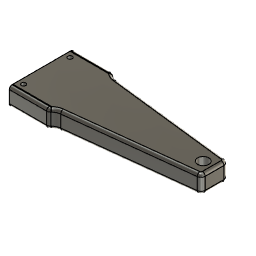
torsionEndPiece_vFINAL v4 (Autodesk Fusion 360 design; units mm, degrees)
Autodesk Fusion 360 part; units mm, degrees
sketch "Sketch1" plane through (0, 0, 0) normal (0, 0, 1) x (1, 0, 0)
  line L0 (0, 0) -> (0, 16)
  line L1 (86.957, 0) -> (0, 0)
  line L2 (0, 16) -> (21.957, 16)
  line L3 (86.957, 0) -> (86.957, 5)
  line L4 (86.957, 5) -> (21.957, 16)
  line L5 (86.957, -5) -> (21.957, -16)
  line L6 (0, -16) -> (21.957, -16)
  line L7 (86.957, 0) -> (86.957, -5)
  line L8 (0, 0) -> (0, -16)
  line L9 (86.957, 5) -> (96.957, 5)
  line L10 (96.957, 5) -> (96.957, -5)
  line L11 (96.957, -5) -> (86.957, -5)
  line L12 (86.957, -5) -> (86.957, 5)
  line L13 (21.957, 16) -> (96.957, 5)
  line L14 (96.957, -5) -> (21.957, -16)
  line L15 (96.957, 5) -> (96.957, 7.35)
  line L16 (96.957, -5) -> (96.957, -7.35)
  line L17 (96.957, 7.35) -> (21.957, 16)
  line L18 (96.957, -7.35) -> (21.957, -16)
  dimension "d1" = 16
  dimension "d20" = 21.957
  dimension "d47" = 65
  dimension "d48" = 5
  dimension "d49" = 10
  dimension "d56" = 2.35
  dimension "d57" = 2.35
  constraint coincident L0.start L1.end
  constraint vertical L0
  constraint perpendicular L0 L1
  constraint perpendicular L0 L2
  constraint perpendicular L1 L3
  constraint symmetric L0.start L1 L8.start
  constraint symmetric L0.end L1 L6.start
  constraint symmetric L3.start L1 L7.start
  constraint symmetric L1 L2.end L5.end
  constraint symmetric L1 L3.end L5.start
  constraint horizontal L9
  constraint vertical L10
  constraint horizontal L11
  constraint vertical L12
  constraint perpendicular L9 L15
  constraint perpendicular L11 L16
  measures "d1" distance of L0.start L0.end
  measures "d20" distance of L0.end L2.end
  measures "d47" horizontal distance of L2.end L3.end
  measures "d48" distance of L1.start L3.end
  measures "d49" distance of L3.end L9.end
  measures "d56" distance of L9.end L15.end
  measures "d57" distance of L10.end L16.end
extrude "Extrude1" add sketch "Sketch1" along normal blind 10 contours L0 L1 L2 L3 L4 L12 | L1 L5 L6 L7 L8 L12
sketch "Sketch2" plane through (0, 0, 0) normal (0, 0, 1) x (1, 0, 0)
  line L0 (0, 16) -> (0, -16)
sketch "Sketch3" plane through (0, 0, 0) normal (-1, 0, 0) x (0, -1, 0)
  line L0 (-16, 0) -> (16, 0)
  line L1 (16, 10) -> (-16, 10)
  line L2 (-16, 8) -> (-11, 8)
  line L3 (-7, 8) -> (-2, 8)
  line L4 (2, 8) -> (7.0009, 8)
  line L5 (-16, 10) -> (-16, 0)
  line L6 (7.0009, 8) -> (7.0009, 2)
  line L7 (7.0009, 2) -> (2, 2)
  line L8 (2, 2) -> (2, 8)
  line L9 (-2, 8) -> (-2, 2)
  line L10 (-2, 2) -> (-7, 2)
  line L11 (-7, 2) -> (-7, 8)
  line L12 (-11, 8) -> (-11, 2)
  line L13 (-11, 2) -> (-16, 2)
  line L14 (16, 8) -> (11, 8)
  line L15 (11, 8) -> (11, 2)
  line L16 (11, 2) -> (16, 2)
  line L17 (16, 2) -> (16, 8)
  dimension "d13" = 5
  dimension "d14" = 5
  dimension "d34" = 4
  dimension "d35" = 4
  constraint perpendicular L4 L6
  constraint perpendicular L6 L7
  constraint perpendicular L3 L9
  constraint perpendicular L9 L10
  constraint perpendicular L2 L12
  constraint coincident L5 L13.end
  constraint perpendicular L5 L13
  constraint horizontal L14
  constraint perpendicular L14 L15
  constraint perpendicular L15 L16
  constraint perpendicular L14 L17
  measures "d13" distance of L2.end L2.start
  measures "d14" distance of L3.start L3.end
  measures "d34" distance of L8 L9
  measures "d35" distance of L11 L12
extrude "Extrude2" cut sketch "Sketch3" against normal blind 20
sketch "Sketch5" plane through (0, 0, 10) normal (0, 0, 1) x (-1, 0, 0)
  line L0 (0, -16) -> (0, 16)
  line L1 (0, 16) -> (-21.957, 16)
  line L2 (-21.957, 16) -> (-86.957, 5)
  line L3 (-86.957, 5) -> (-86.957, -5)
  line L4 (-86.957, -5) -> (-21.957, -16)
  line L5 (-21.957, -16) -> (0, -16)
  circle A0 centre (-3, -13) radius 1
  circle A1 centre (-3, 13) radius 1
  dimension "d24" = 2
  dimension "d25" = 2
  dimension "d26" = 3
  dimension "d27" = 3
  dimension "d28" = 3
  dimension "d29" = 3
  measures "d24" diameter of A0
  measures "d25" diameter of A1
  measures "d26" distance of L0 A0.centre
  measures "d27" distance of L5 A0.centre
  measures "d28" distance of L0 A1.centre
  measures "d29" distance of L1 A1.centre
sketch "Sketch6" plane through (0, 0, 0) normal (-1, 0, 0) x (0, -1, 0)
  line L0 (-11, 2) -> (-16, 2)
  line L1 (-16, 2) -> (-16, 0)
  line L2 (-16, 0) -> (16, 0)
  line L3 (16, 0) -> (16, 2)
  line L4 (16, 2) -> (11, 2)
  line L5 (11, 2) -> (11, 8)
  line L6 (11, 8) -> (16, 8)
  line L7 (16, 8) -> (16, 10)
  line L8 (16, 10) -> (-16, 10)
  line L9 (-16, 10) -> (-16, 8)
  line L10 (-16, 8) -> (-11, 8)
  line L11 (-11, 8) -> (-11, 2)
  line L12 (-2, 8) -> (-2, 2)
  line L13 (-2, 2) -> (-7, 2)
  line L14 (-7, 2) -> (-7, 8)
  line L15 (-7, 8) -> (-2, 8)
  line L16 (7.0009, 8) -> (7.0009, 2)
  line L17 (7.0009, 2) -> (2, 2)
  line L18 (2, 2) -> (2, 8)
  line L19 (2, 8) -> (7.0009, 8)
  line L20 (16, 0) -> (18, 0)
  line L21 (18, 0) -> (18, 10)
  line L22 (18, 10) -> (16, 10)
  line L23 (16, 2) -> (16, 8)
  line L24 (16, 2) -> (16, 0)
  line L25 (16, 8) -> (16, 10)
  line L26 (-16, 0) -> (-18, 0)
  line L27 (-18, 0) -> (-18, 10)
  line L28 (-18, 10) -> (-16, 10)
  line L29 (-16, 8) -> (-16, 2)
  line L30 (-16, 2) -> (-16, 0)
  line L31 (-16, 8) -> (-16, 10)
  dimension "d36" = 2
  dimension "d37" = 10
  constraint coincident L2.end L3.start
  constraint perpendicular L3 L20
  constraint perpendicular L20 L21
  constraint coincident L7.end L8.start
  constraint coincident L3.end L4.start
  constraint coincident L6.end L7.start
  constraint coincident L1.end L2.start
  constraint perpendicular L1 L26
  constraint perpendicular L26 L27
  constraint coincident L8.end L9.start
  constraint coincident L9.end L10.start
  constraint coincident L0.end L1.start
  measures "d36" distance of L2.end L20.end
  measures "d37" distance of L20.end L21.end
extrude "Extrude4" add sketch "Sketch6" against normal up to surface (21.957 mm away) contours L1 L9 L26 L27 L28 L29 L30 L31 | L3 L7 L20 L21 L22 L23 L24 L25
sketch "Sketch7" plane through (0, 0, 0) normal (-1, 0, 0) x (0, -1, 0)
  line L0 (-16, 8) -> (-11, 8)
  line L1 (-11, 8) -> (-11, 2)
  line L2 (-11, 2) -> (-16, 2)
  line L3 (-16, 2) -> (-16, 8)
  line L4 (16, 2) -> (11, 2)
  line L5 (11, 2) -> (11, 8)
  line L6 (11, 8) -> (16, 8)
  line L7 (16, 8) -> (16, 2)
  line L8 (-16, 10) -> (-18, 10)
  line L9 (-18, 10) -> (-18, 0)
  line L10 (-18, 0) -> (16, 0)
  line L11 (16, 0) -> (18, 0)
  line L12 (18, 0) -> (18, 10)
  line L13 (18, 10) -> (16, 10)
  line L14 (16, 10) -> (-16, 10)
  line L15 (-2, 8) -> (-2, 2)
  line L16 (-2, 2) -> (-7, 2)
  line L17 (-7, 2) -> (-7, 8)
  line L18 (-7, 8) -> (-2, 8)
  line L19 (7.0009, 8) -> (7.0009, 2)
  line L20 (7.0009, 2) -> (2, 2)
  line L21 (2, 2) -> (2, 8)
  line L22 (2, 8) -> (7.0009, 8)
  line L23 (16, 2) -> (-16, 2)
  line L24 (-16, 8) -> (16, 8)
  line L25 (16, 2) -> (16, 8)
  line L26 (-16, 2) -> (-16, 8)
  constraint coincident L4.start L7.end
  constraint coincident L2.end L3.start
  constraint coincident L0.start L3.end
  constraint coincident L6.end L7.start
sketch "Sketch8" plane through (0, 0, 0) normal (-1, 0, 0) x (0, -1, 0)
  line L0 (-16, 8) -> (-11, 8)
  line L1 (-11, 8) -> (-11, 2)
  line L2 (-11, 2) -> (-16, 2)
  line L3 (-16, 2) -> (-16, 8)
  line L4 (16, 2) -> (11, 2)
  line L5 (11, 2) -> (11, 8)
  line L6 (11, 8) -> (16, 8)
  line L7 (16, 8) -> (16, 2)
  line L8 (-16, 10) -> (-18, 10)
  line L9 (-18, 10) -> (-18, 0)
  line L10 (-18, 0) -> (16, 0)
  line L11 (16, 0) -> (18, 0)
  line L12 (18, 0) -> (18, 10)
  line L13 (18, 10) -> (16, 10)
  line L14 (16, 10) -> (-16, 10)
  line L15 (-2, 8) -> (-2, 2)
  line L16 (-2, 2) -> (-7, 2)
  line L17 (-7, 2) -> (-7, 8)
  line L18 (-7, 8) -> (-2, 8)
  line L19 (7.0009, 8) -> (7.0009, 2)
  line L20 (7.0009, 2) -> (2, 2)
  line L21 (2, 2) -> (2, 8)
  line L22 (2, 8) -> (7.0009, 8)
  line L23 (11, 2) -> (7.0009, 2)
  line L24 (11, 8) -> (7.0009, 8)
  line L25 (2, 2) -> (-2, 2)
  line L26 (-2, 8) -> (2, 8)
  line L27 (-7, 2) -> (-11, 2)
  line L28 (-11, 8) -> (-7, 8)
  constraint coincident L4.end L5.start
  constraint coincident L19.end L20.start
  constraint coincident L5.end L6.start
  constraint coincident L19.start L22.end
  constraint coincident L20.end L21.start
  constraint coincident L15.end L16.start
  constraint coincident L15.start L18.end
  constraint coincident L21.end L22.start
  constraint coincident L16.end L17.start
  constraint coincident L1.end L2.start
  constraint coincident L0.end L1.start
  constraint coincident L17.end L18.start
extrude "Extrude6" cut sketch "Sketch8" against normal blind 5 contours L1 L17 L27 L28 | L15 L21 L25 L26 | L5 L19 L23 L24
extrude "Extrude7" cut sketch "Sketch5" against normal up to surface (10 mm away) contours A0 | A1
extrude "Extrude8" add sketch "Sketch1" along normal blind 10 contours L3 L7 L9 L10 L11 L12 | L4 L9 L13 | L5 L11 L14
sketch "Sketch9" plane through (0, 0, 10) normal (0, 0, 1) x (-1, 0, 0)
  circle A0 centre (-3, -13) radius 1
  circle A1 centre (-3, 13) radius 1
  line L0 (0, -16) -> (0, 16)
  line L1 (0, 16) -> (-21.957, 16)
  line L2 (-21.957, 16) -> (-96.957, 5)
  line L3 (-96.957, 5) -> (-96.957, -5)
  line L4 (-96.957, -5) -> (-21.957, -16)
  line L5 (-21.957, -16) -> (0, -16)
  line L6 (-96.957, 0) -> (-90.607, 0)
  circle A2 centre (-90.607, 0) radius 3.175
  dimension "d52" = 6.35
  dimension "d53" = 6.35
  constraint midpoint L3 L6.start
  constraint perpendicular L3 L6
  constraint coincident L6.end A2.centre
  measures "d52" distance of L6.start L6.end
  measures "d53" diameter of A2
extrude "Extrude9" cut sketch "Sketch9" against normal blind 45 contours A2
extrude "Extrude10" add sketch "Sketch1" along normal blind 10 contours L13 L15 L17 | L14 L16 L18
fillet "Fillet1" radius 2.3813 2 edges at (96.957, -7.35, 5) (96.957, 7.35, 5)
fillet "Fillet2" radius 1 6 edges at (5, -11, 5) (5, -7.0009, 5) (5, -2, 5) (5, 2, 5) (5, 7, 5) (5, 11, 5)
chamfer "Chamfer1" distance 0.5 angle 45 14 edges at (0, -4.5005, 8) (0, -9.0005, 8) (0, -13.5, 8) (0, 13.5, 8) (0, 9, 8) (0, 4.5, 8) (0, 0, 8) (0, 16, 5) (0, 9, 2) (0, -13.5, 2) (0, -9.0005, 2) (0, -4.5005, 2) (0, 0, 2) (0, -16, 5)
fillet "Fillet3" radius 6.35 2 edges at (21.957, -16, 5) (21.957, 16, 5)
fillet "Fillet4" radius 2.3813 2 edges at (21.957, -18, 5) (21.957, 18, 5)
fillet "Fillet5" radius 1.5875 12 edges at (10.4397, -18, 10) (21.7883, -17.8197, 10) (24.286, -16.0842, 10) (60.5806, -11.5454, 10) (96.3534, -6.812, 10) (96.957, 0, 10) (96.3534, 6.812, 10) (60.5806, 11.5454, 10) (24.2835, 16.0854, 10) (22.2754, 17.5478, 10) (21.4334, 17.9347, 10) (10.4397, 18, 10)
fillet "Fillet6" radius 1.5875 11 edges at (10.4397, 18, 0) (21.7883, 17.8197, 0) (24.2835, 16.0854, 0) (60.5806, 11.5454, 0) (96.3534, 6.812, 0) (96.957, 0, 0) (96.3534, -6.812, 0) (60.5806, -11.5454, 0) (24.2818, -16.0862, 0) (21.7883, -17.8197, 0) (10.4397, -18, 0)
move_face "OffsetFaces1" offset -0.25 2 faces at (2.005, -12.9004, 8.6667) (2.005, 13.0996, 9.3333)
move_face "OffsetFaces2" offset -0.25 2 faces at (2.005, 13.0996, 1.3333) (2.005, -12.9004, 1.3333)
